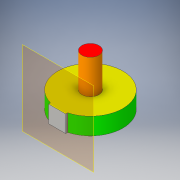
# Autodesk Inventor part: T100 rough draft
Saved by Autodesk Inventor 2016 (Build 200138000, 138)
## iProperties
Created: 2017-02-01
Part Number: T100 rough draft
Material: Generic
Document SubType Name: Modeling
Designer: student1
Density: 1 g/cm^3
Appearance: Default
Author: student1
Autodesk Inventor part; units mm, degrees
ref_plane "YZ Plane" through (0, 0, 0) normal (1, 0, 0) x (0, 1, 0)
ref_plane "XZ Plane" through (0, 0, 0) normal (0, 1, 0) x (-1, 0, 0)
sketch "Sketch1" plane through (0, 0, 0) normal (0, 1, 0) x (-1, 0, 0)
  circle A0 centre (0, 0) radius 48.26
  dimension "d0" = 96.52
  constraints: 1 centre point, 1 coincident
  measures "d0" diameter of A0
extrude "Extrusion1" add sketch "Sketch1" along normal blind 25.4
sketch "Sketch2" plane through (0, 25.4, 0) normal (0, 1, 0) x (1, 0, 0)
  circle A0 centre (0, 0) radius 12.7
  dimension "d3" = 25.4
  constraints: 1 centre point, 1 coincident
  measures "d3" diameter of A0
extrude "Extrusion2" add sketch "Sketch2" along normal blind 50.8
sketch "Sketch3" plane through (0, 0, 0) normal (0, -1, 0) x (1, 0, 0)
  circle A0 centre (0, 0) radius 12.7 projected
  circle A1 centre (0, 0) radius 12.7
  constraints: 1 centre point, 1 coincident
extrude "Extrusion3" add sketch "Sketch3" along normal blind 25.4
ref_plane "Work Plane1" through (0, 0, 48.26) normal (0, 0, 1) x (1, 0, 0)
sketch "Sketch4" plane through (0, 0, 48.26) normal (0, 0, 1) x (1, 0, 0)
  line L0 (0, 0) -> (0, 25.4)
  line L1 (0, 0) -> (12.7, 0)
  line L2 (0, 0) -> (-12.7, 0)
  line L3 (12.7, 0) -> (12.7, 25.4)
  line L4 (12.7, 25.4) -> (-12.7, 25.4)
  line L5 (-12.7, 25.4) -> (-12.7, 0)
  line L6 (-48.26, 0) -> (48.26, 0) projected
  dimension "d9" = 12.7
  dimension "d10" = 25.4
  dimension "d11" = 12.7
  constraints: 12 end point, 1 perpendicular
  measures "d9" distance of L0.start L1.end
  measures "d10" distance of L3.end L4.end
  measures "d11" distance of L0.start L2.end
extrude "Extrusion4" add sketch "Sketch4" along normal blind 1.27 and the other way blind 12.7
body "Solid1"
